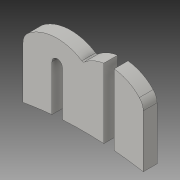
# Autodesk Inventor part: Bikair_Logo
Saved by Autodesk Inventor 2016 (Build 200138000, 138)
## iProperties
Created: 2015-05-14
Part Number: Bikair_Logo
Material: Generic
Document SubType Name: Modeling
Designer: Yann
Density: 1 g/cm^3
Appearance: Default
Author: Yann
Autodesk Inventor part; units mm, degrees
ref_plane "YZ Plane" through (0, 0, 0) normal (1, 0, 0) x (0, 1, 0)
ref_plane "XZ Plane" through (0, 0, 0) normal (0, 1, 0) x (-1, 0, 0)
ref_plane "XY Plane" through (0, 0, 0) normal (0, 0, 1) x (1, 0, 0)
sketch "Sketch1" plane through (0, 0, 0) normal (0, 0, 1) x (1, 0, 0)
  line L0 (0, 24.8103) -> (0, -128.2631) construction
  line L1 (-69.1744, 0) -> (69.1744, 0) construction
  circle A0 centre (0, -56.9852) radius 49.4103 construction
  line L2 (-8.7, -8.3468) -> (-8.7, -0.8651)
  line L3 (-4.5, -7.7802) -> (-4.5, -1.144)
  line L4 (-3, -7.666) -> (-3, -1.144)
  line L5 (4.5, -7.7802) -> (4.5, 2.4506)
  line L6 (8.7, -8.3468) -> (8.7, -0.711)
  line L7 (3, -7.666) -> (3, 2.4116)
  line L8 (-3, -1.144) -> (-4.5, -1.144) construction
  arc A1 (-3, -1.144) -> (-4.5, -1.144) centre (-3.75, -1.144) ccw
  arc A2 (-4.5, -7.7802) -> (-8.7, -8.3468) centre (0, -56.9852) ccw
  arc A3 (3, -7.666) -> (-3, -7.666) centre (0, -56.9852) ccw
  arc A4 (8.7, -8.3468) -> (4.5, -7.7802) centre (0, -56.9852) ccw
  arc A5 (-0.184, 1.1203) -> (-7.943, 0.7018) centre (-3.7683, -4.5606) ccw
  arc A6 (8.7, 0) -> (0, 1) centre (3.9019, -3.3989) ccw construction
  arc A7 (-7.943, 0.7018) -> (-8.7, -0.8651) centre (-6.7, -0.8651) ccw
  arc A8 (3, 2.4116) -> (0.1667, 1.1424) centre (3.9019, -3.3989) ccw
  arc A9 (8.1423, 0.6746) -> (4.5, 2.4506) centre (3.9019, -3.3989) ccw
  arc A10 (8.7, -0.711) -> (8.1423, 0.6746) centre (6.7, -0.711) ccw
  arc A11 (-0.184, 1.1203) -> (0.1667, 1.1424) centre (-0.0239, 1.3741) ccw
  point P0 (-8.7, 0)
  point P1 (8.7, 0)
  dimension "d0" = 4.2
  dimension "d1" = 1.5
  dimension "d2" = 3
  dimension "d3" = 2
  dimension "d5" = 1
  dimension "d6" = 2
  dimension "d7" = 0.3
  constraints: 35 point on circle, 14 end point, 12 centre point, 7 point on line, 7 tangent, 3 coincident, 3 perpendicular, 3 vertical, 2 concentric, 1 horizontal, 1 midpoint, 3 other
  measures "d0" distance between parallel lines of L3 L2
  measures "d1" distance between parallel lines of L3 L4
  measures "d2" distance between parallel lines of L4 L0
  measures "d3" radius of A7
  measures "d5" distance from line of A6.end L1
  measures "d6" radius of A10
  measures "d7" radius of A11
extrude "Extrusion1" add sketch "Sketch1" along normal mid plane 2
equation "\"d6\" = d3"
body "Solid1"
